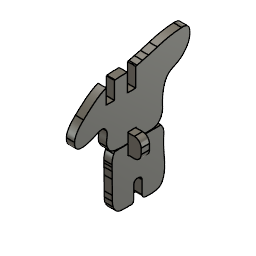
MORFY Test1 (Autodesk Fusion 360 design; units mm, degrees)
Autodesk Fusion 360 part; units mm, degrees
note: some values were not read from the file. Chosen so that the rebuilt part matches the saved one: that a step has no effect; which pieces of a blend or face edit are solid. Set by a fixed rule: which sketch regions a step uses.
sketch "Sketch7" plane through (0, 0, 0) normal (1, 0, 0) x (0, 0, -1)
  line L0 (0, 0) -> (80, 0)
  line L1 (80, 0) -> (80, 80)
  line L2 (80, 80) -> (0, 80)
  line L3 (0, 80) -> (0, 0)
  line L4 (34, 0) -> (46, 0)
  line L5 (46, 0) -> (46, 30)
  line L6 (46, 30) -> (34, 30)
  line L7 (34, 30) -> (34, 0)
  line L8 (25.6401, 80) -> (37.6401, 80)
  line L9 (37.6401, 80) -> (37.6401, 65)
  line L10 (37.6401, 65) -> (25.6401, 65)
  line L11 (25.6401, 65) -> (25.6401, 80)
  line L12 (-92.3642, 110) -> (183.4543, 110)
  line L13 (183.4543, 110) -> (183.4543, 204.562)
  line L14 (-92.3642, 204.562) -> (-92.3642, 110)
  line L15 (25.6401, 110) -> (37.6401, 110)
  line L16 (37.6401, 110) -> (37.6401, 125)
  line L17 (37.6401, 125) -> (25.6401, 125)
  line L18 (25.6401, 125) -> (25.6401, 110)
  line L19 (24.6547, 204.562) -> (36.6547, 204.562)
  line L20 (36.6547, 204.562) -> (36.6547, 174.562)
  line L21 (36.6547, 174.562) -> (24.6547, 174.562)
  line L22 (24.6547, 174.562) -> (24.6547, 204.562)
  line L23 (-6.0953, 204.562) -> (5.9047, 204.562)
  line L24 (5.9047, 204.562) -> (5.9047, 174.562)
  line L25 (5.9047, 174.562) -> (-6.0953, 174.562)
  line L26 (-6.0953, 174.562) -> (-6.0953, 204.562)
  spline S0 degree 3 poles (115.5, 205.2559) (115.6659, 197.3379) (111.8252, 191.1596) (109.8122, 188.2657) knots 0 0 0 0 1 1 1 1
  spline S1 degree 3 poles (109.8122, 188.2657) (98.6392, 172.2077) (87.6076, 176.7145) (80.9024, 164.5312) knots 0 0 0 0 1 1 1 1
  spline S2 degree 3 poles (80.9024, 164.5312) (74.7119, 153.2655) (75.727, 134.0915) (75.7904, 133.0545) knots 0 0 0 0 1 1 1 1
  spline S3 degree 3 poles (75.7904, 133.0545) (75.8978, 131.2756) (76.3565, 125.3731) (73.2991, 119.5316) knots 0 0 0 0 1 1 1 1
  spline S4 degree 3 poles (73.2991, 119.5316) (72.5427, 118.0871) (71.0421, 115.3006) (67.9603, 113.3119) knots 0 0 0 0 1 1 1 1
  spline S5 degree 3 poles (67.9603, 113.3119) (64.7418, 111.2354) (61.499, 111.1281) (58.0561, 111.0597) knots 0 0 0 0 1 1 1 1
  spline S6 degree 3 poles (58.0561, 111.0597) (49.4695, 110.8865) (42.9277, 110.9475) (39.9264, 110.9377) knots 0 0 0 0 1 1 1 1
  spline S7 degree 2 poles (39.9264, 110.9377) (27.9262, 110.9036) (20.4889, 110.5059) knots 0 0 0 1 1 1
  spline S8 degree 3 poles (20.4889, 110.5059) (17.9976, 110.3741) (13.2956, 110.091) (7.4053, 111.2379) knots 0 0 0 0 1 1 1 1
  spline S9 degree 3 poles (7.4053, 111.2379) (3.4206, 112.0187) (1.4808, 112.9459) (-0.0686, 114.1879) knots 0 0 0 0 1 1 1 1
  spline S10 degree 3 poles (-0.0686, 114.1879) (-2.5477, 116.1692) (-3.6189, 118.7069) (-4.5559, 121.0054) knots 0 0 0 0 1 1 1 1
  spline S11 degree 3 poles (-4.5559, 121.0054) (-8.072, 129.6262) (-2.2427, 134.6698) (-5.8223, 142.2779) knots 0 0 0 0 1 1 1 1
  spline S12 degree 3 poles (-5.8223, 142.2779) (-7.4059, 145.6476) (-9.3409, 146.5626) (-9.802, 146.7627) knots 0 0 0 0 1 1 1 1
  spline S13 degree 3 poles (-9.802, 146.7627) (-12.469, 147.9266) (-15.2165, 146.7749) (-18.3618, 145.4866) knots 0 0 0 0 1 1 1 1
  spline S14 degree 3 poles (-18.3618, 145.4866) (-23.1907, 143.5077) (-33.8025, 138.7276) (-40.0783, 138.5177) knots 0 0 0 0 1 1 1 1
  spline S15 degree 3 poles (-40.0783, 138.5177) (-45.7417, 138.3299) (-47.7962, 139.8647) (-48.3135, 140.2258) knots 0 0 0 0 1 1 1 1
  spline S16 degree 3 poles (-48.3135, 140.2258) (-51.4856, 142.4828) (-52.4372, 146.8408) (-52.1005, 150.7181) knots 0 0 0 0 1 1 1 1
  spline S17 degree 3 poles (-52.1005, 150.7181) (-51.4661, 158.0382) (-47.3887, 164.4727) (-38.9095, 172.359) knots 0 0 0 0 1 1 1 1
  spline S18 degree 3 poles (-38.9095, 172.359) (-25.0036, 185.323) (-12.4788, 196.9767) (6.8319, 199.8438) knots 0 0 0 0 1 1 1 1
  spline S19 degree 3 poles (6.8319, 199.8438) (17.8292, 201.4835) (23.7268, 199.1899) (38.6039, 202.462) knots 0 0 0 0 1 1 1 1
  spline S20 degree 3 poles (38.6039, 202.462) (45.0774, 203.8845) (48.2251, 205.2559) (55.4232, 206.7614) knots 0 0 0 0 1 1 1 1
  spline S21 degree 2 poles (55.4232, 206.7614) (62.0968, 208.8598) (68.1335, 210.685) knots 0 0 0 1 1 1
  spline S22 degree 2 poles (68.1335, 210.685) (85.6678, 216.446) (103.4778, 217.4562) knots 0 0 0 1 1 1
  spline S23 degree 3 poles (103.4778, 217.4562) (106.035, 217.6026) (109.0777, 217.6221) (111.713, 215.7481) knots 0 0 0 0 1 1 1 1
  spline S24 degree 3 poles (111.713, 215.7481) (115.4658, 213.0811) (115.4512, 207.569) (115.5, 205.2559) knots 0 0 0 0 1 1 1 1
  line L27 (183.4543, 204.562) -> (46.6766, 204.562)
  line L28 (36.6547, 204.562) -> (-92.3642, 204.562)
  line L29 (36.6547, 204.562) -> (118.2693, 237.026)
  line L30 (118.2693, 237.026) -> (183.4543, 204.562)
  dimension "d65" = 80
  dimension "d66" = 12
  dimension "d67" = 30
  dimension "d68" = 80
  dimension "d69" = 12
  dimension "d70" = 15
  dimension "d74" = 30
  dimension "d77" = 12
  dimension "d78" = 15
  dimension "d79" = 12
  dimension "d80" = 12
  dimension "d81" = 30
  dimension "d82" = 30
  dimension "d85" = 18.75
  constraint horizontal L0
  constraint vertical L1
  constraint horizontal L2
  constraint vertical L3
  constraint coincident L0.start L3.end
  constraint horizontal L4
  constraint vertical L5
  constraint horizontal L6
  constraint vertical L7
  constraint coincident L0 L4.start
  constraint midpoint L0 L4
  constraint horizontal L8
  constraint vertical L9
  constraint horizontal L10
  constraint vertical L11
  constraint coincident L2 L8.start
  constraint horizontal L12
  constraint vertical L13
  constraint horizontal L27
  constraint vertical L14
  constraint horizontal L15
  constraint vertical L16
  constraint horizontal L17
  constraint vertical L18
  constraint coincident L12 L15.start
  constraint horizontal L19
  constraint vertical L20
  constraint horizontal L21
  constraint vertical L22
  constraint coincident L19.start L28
  constraint horizontal L23
  constraint vertical L24
  constraint horizontal L25
  constraint vertical L26
  constraint coincident L23.start L28
  constraint collinear L11 L18
  constraint coincident S20 L27.end
  constraint collinear L27 L28
  measures "d65" distance of L0.end L1.end
  measures "d66" distance of L5.end L6.end
  measures "d67" distance of L4.end L5.end
  measures "d68" distance of L1.end L2.end
  measures "d69" distance of L9.end L10.end
  measures "d70" distance of L8.start L10.end
  measures "d74" distance of L2 L12
  measures "d77" distance of L16.end L17.end
  measures "d78" distance of L15.end L16.end
  measures "d79" distance of L24.end L25.end
  measures "d80" distance of L20.end L21.end
  measures "d81" distance of L23.start L25.end
  measures "d82" distance of L19.end L20.end
  measures "d85" distance of L22 L24
extrude "Extrude10" add sketch "Sketch7" along normal blind 12 contours L0 L1 L2 L3 L5 L6 L7 L9 L10 L11 makes body 1
extrude "Extrude11" add sketch "Sketch7" along normal blind 12 separate body contours L12 L14 L18 L26 S7 S8 S9 S10 S11 S12 S13 S14 S15 S16 S17 S18 L28 | L12 L13 L16 S0 S1 S2 S3 S4 S5 S6 S7 L27 | L16 L17 L18 L20 L21 L22 L24 L25 L26 S0 S1 S2 S3 S4 S5 S6 S7 S8 S9 S10 S11 S12 S13 S14 S15 S16 S17 S18 S19 S20 L27 | L22 L24 S18 S19 L28 | L20 S0 S19 S20 S21 S22 S23 S24 L27 L29 L30 | S0 S20 S21 S22 S23 S24 L27 makes body 2
extrude "Extrude14" cut sketch "Sketch7" along normal up to surface (12 mm away) contours L16 L17 L18 L20 L21 L22 L24 L25 L26 S0 S1 S2 S3 S4 S5 S6 S7 S8 S9 S10 S11 S12 S13 S14 S15 S16 S17 S18 S19 S20 L27 | S0 S20 S21 S22 S23 S24 L27 keep common part bodies 2
move_body "Move3" bodies 2 to x (1, 0, 0) y (0, 1, 0) z (0, 0, 1) at (0, -30, 0)
sketch "Sketch8" plane through (0, 0, 0) normal (0, 0, 1) x (1, 0, 0)
  line L0 (-19, 94) -> (31, 94)
  line L1 (31, 94) -> (31, 66)
  line L2 (31, 66) -> (-19, 66)
  line L3 (-19, 66) -> (-19, 94)
  line L4 (0, 95) -> (12, 95)
  line L5 (0, 65) -> (12, 65)
  line L6 (6, 95) -> (6, 65) construction
  line L7 (0, 80) -> (12, 80)
  line L8 (-19, 80) -> (31, 80) construction
  line L9 (6, 94) -> (6, 66) construction
  dimension "d90" = 30
  dimension "d91" = 28
  dimension "d93" = 50
  constraint horizontal L0
  constraint vertical L1
  constraint horizontal L2
  constraint vertical L3
  constraint midpoint L4 L6.start
  constraint midpoint L5 L6.end
  constraint midpoint L3 L8.start
  constraint midpoint L1 L8.end
  constraint collinear L7 L8
  constraint midpoint L0 L9.start
  constraint midpoint L2 L9.end
  constraint collinear L6 L9
  measures "d90" distance of L4 L5
  measures "d91" distance of L0.end L1.end
  measures "d93" distance of L1.end L2.end
extrude "Extrude12" add sketch "Sketch8" along normal blind 12 from surface at -37.6401 separate body makes body 3
fillet "Fillet5" [no effect]
sketch "Sketch9" plane through (0, 0, 0) normal (-1, 0, 0) x (0, 0, 1)
  line L0 (-80, 0) -> (-46, 0)
  line L1 (-46, 0) -> (-46, 30)
  line L2 (-46, 30) -> (-34, 30)
  line L3 (-34, 30) -> (-34, 0)
  line L4 (-34, 0) -> (0, 0)
  line L5 (0, 0) -> (0, 80)
  line L6 (0, 80) -> (-25.6401, 80)
  line L7 (-25.6401, 80) -> (-25.6401, 65)
  line L8 (-25.6401, 65) -> (-37.6401, 65)
  line L9 (-37.6401, 65) -> (-37.6401, 80)
  line L10 (-37.6401, 80) -> (-80, 80)
  line L11 (-80, 80) -> (-80, 0)
sketch "Sketch10" plane through (0, 0, 0) normal (-1, 0, 0) x (0, 0, 1)
  line L0 (-34, 0) -> (0, 0)
  line L1 (0, 0) -> (0, 80)
  line L2 (0, 80) -> (-25.6401, 80)
  line L3 (-25.6401, 80) -> (-25.6401, 65)
  line L4 (-25.6401, 65) -> (-37.6401, 65)
  line L5 (-37.6401, 65) -> (-37.6401, 80)
  line L6 (-37.6401, 80) -> (-80, 80)
  line L7 (-80, 80) -> (-80, 0)
  line L8 (-80, 0) -> (-46, 0)
  line L9 (-46, 0) -> (-46, 30)
  line L10 (-46, 30) -> (-34, 30)
  line L11 (-34, 30) -> (-34, 0)
  spline S0 degree 3 poles (-73.7036, 81.706) (-75.3725, 79.425) (-76.9127, 77.0041) (-77.8839, 74.3392) knots 0 0 0 0 1 1 1 1
  arc A0 (-78.9408, 68.1331) -> (-77.8839, 74.3392) centre (-61.374, 68.3344) cw
  spline S1 degree 3 poles (-78.9408, 68.1331) (-78.9137, 65.6625) (-78.6043, 63.1986) (-78.4891, 60.7302) knots 0 0 0 0 1 1 1 1
  spline S2 degree 3 poles (-78.4891, 60.7302) (-78.3988, 58.9235) (-78.3988, 57.1326) (-78.4394, 55.3327) knots 0 0 0 0 1 1 1 1
  spline S3 degree 3 poles (-78.4394, 55.3327) (-78.5614, 50.0842) (-78.7533, 44.8086) (-79.196, 39.576) knots 0 0 0 0 1 1 1 1
  spline S4 degree 3 poles (-79.196, 39.576) (-79.4376, 36.7033) (-79.8509, 33.851) (-79.9548, 30.9648) knots 0 0 0 0 1 1 1 1
  spline S5 degree 3 poles (-79.9548, 30.9648) (-80.1422, 25.8428) (-80.0587, 20.6146) (-79.0198, 15.5784) knots 0 0 0 0 1 1 1 1
  arc A1 (-77.3102, 9.8715) -> (-79.0198, 15.5784) centre (-45.9875, 22.3642) cw
  spline S6 degree 3 poles (-77.3102, 9.8715) (-76.3436, 7.4505) (-75.2325, 5.0634) (-73.2158, 3.3222) knots 0 0 0 0 1 1 1 1
  spline S7 degree 3 poles (-73.2158, 3.3222) (-71.5762, 1.913) (-69.6024, 1.118) (-67.5179, 0.5941) knots 0 0 0 0 1 1 1 1
  arc A2 (-58.5002, -0.5983) -> (-67.5179, 0.5941) centre (-57.5378, 41.3739) cw
  spline S8 degree 3 poles (-58.5002, -0.5983) (-55.964, -0.6706) (-53.4324, -0.4809) (-50.8985, -0.386) knots 0 0 0 0 1 1 1 1
  spline S9 degree 3 poles (-50.8985, -0.386) (-45.9459, -0.2008) (-40.9865, -0.1195) (-36.0271, -0.1015) knots 0 0 0 0 1 1 1 1
  spline S10 degree 3 poles (-36.0271, -0.1015) (-31.4674, -0.0834) (-26.9077, -0.1015) (-22.3458, -0.0473) knots 0 0 0 0 1 1 1 1
  spline S11 degree 3 poles (-22.3458, -0.0473) (-19.349, -0.0066) (-16.2188, -0.1579) (-13.2739, 0.5105) knots 0 0 0 0 1 1 1 1
  arc A3 (-6.1781, 4.9618) -> (-13.2739, 0.5105) centre (-16.1754, 13.0173) cw
  spline S12 degree 3 poles (-6.1781, 4.9618) (-2.9667, 8.9072) (-1.7088, 14.0224) (-1.7223, 19.0315) knots 0 0 0 0 1 1 1 1
  spline S13 degree 3 poles (-1.7223, 19.0315) (-1.7381, 25.0952) (-1.6387, 31.159) (-1.5755, 37.2227) knots 0 0 0 0 1 1 1 1
  line L12 (-1.5755, 37.2227) -> (-1.3632, 57.7853)
  spline S14 degree 3 poles (-1.3632, 57.7853) (-1.3452, 59.4271) (-1.3836, 61.078) (-1.2864, 62.7153) knots 0 0 0 0 1 1 1 1
  spline S15 degree 3 poles (-1.2864, 62.7153) (-1.2187, 63.8445) (-1.1938, 64.9985) (-1.2187, 66.139) knots 0 0 0 0 1 1 1 1
  arc A4 (-1.9888, 72.7448) -> (-1.2187, 66.139) centre (-34.5458, 65.6015) cw
  spline S16 degree 3 poles (-1.9888, 72.7448) (-2.8989, 76.8211) (-4.8231, 80.7755) (-8.0684, 83.5082) knots 0 0 0 0 1 1 1 1
  arc A5 (-13.9017, 86.7015) -> (-8.0684, 83.5082) centre (-19.127, 70.2317) cw
  arc A6 (-17.8675, 87.6433) -> (-13.9017, 86.7015) centre (-23.2006, 56.3645) cw
  arc A7 (-22.7636, 88.2463) -> (-17.8675, 87.6433) centre (-25.5631, 45.3357) cw
  spline S17 degree 3 poles (-22.7636, 88.2463) (-25.9728, 88.4721) (-29.1887, 88.4427) (-32.4024, 88.4721) knots 0 0 0 0 1 1 1 1
  spline S18 degree 3 poles (-32.4024, 88.4721) (-35.3609, 88.4992) (-38.3193, 88.5647) (-41.2778, 88.6189) knots 0 0 0 0 1 1 1 1
  spline S19 degree 3 poles (-41.2778, 88.6189) (-46.4111, 88.7137) (-51.5715, 88.8199) (-56.689, 88.3366) knots 0 0 0 0 1 1 1 1
  spline S20 degree 3 poles (-56.689, 88.3366) (-60.9054, 87.9369) (-65.1669, 87.1193) (-68.961, 85.15) knots 0 0 0 0 1 1 1 1
  arc A8 (-73.6133, 81.8212) -> (-68.961, 85.15) centre (-59.5693, 67.1093) cw
  spline S21 degree 3 poles (-73.6133, 81.8212) (-74.1327, 81.3176) (-73.3332, 80.5204) (-72.8002, 81.024) knots 0 0 0 0 1 1 1 1
  spline S22 degree 3 poles (-72.8002, 81.024) (-69.966, 83.7363) (-66.3774, 85.3601) (-62.5879, 86.2634) knots 0 0 0 0 1 1 1 1
  spline S23 degree 3 poles (-62.5879, 86.2634) (-58.1343, 87.3248) (-53.5069, 87.51) (-48.9473, 87.5484) knots 0 0 0 0 1 1 1 1
  spline S24 degree 3 poles (-48.9473, 87.5484) (-43.3781, 87.5959) (-37.8134, 87.3813) (-32.2465, 87.3361) knots 0 0 0 0 1 1 1 1
  spline S25 degree 3 poles (-32.2465, 87.3361) (-29.0555, 87.309) (-25.8644, 87.3361) (-22.6801, 87.1103) knots 0 0 0 0 1 1 1 1
  arc A9 (-22.6801, 87.1103) -> (-17.9217, 86.5073) centre (-25.2821, 47.5002) cw
  arc A10 (-17.9217, 86.5073) -> (-14.0824, 85.5859) centre (-23.408, 55.1885) cw
  arc A11 (-14.0824, 85.5859) -> (-4.9315, 77.7267) centre (-19.0277, 70.5707) cw
  spline S26 degree 3 poles (-4.9315, 77.7267) (-2.9825, 73.9507) (-2.3411, 69.5966) (-2.3276, 65.3915) knots 0 0 0 0 1 1 1 1
  spline S27 degree 3 poles (-2.3276, 65.3915) (-2.3276, 64.2239) (-2.4247, 63.0653) (-2.4382, 61.9023) knots 0 0 0 0 1 1 1 1
  line L13 (-2.4382, 61.9023) -> (-2.4902, 56.8255)
  line L14 (-2.4902, 56.8255) -> (-2.594, 46.7644)
  line L15 (-2.594, 46.7644) -> (-2.8041, 26.5496)
  spline S28 degree 2 poles (-2.8041, 26.5496) (-2.8447, 22.742) (-2.8402, 18.9366) knots 0 0 0 1 1 1
  arc A12 (-2.8402, 18.9366) -> (-3.9423, 11.4366) centre (-26.4737, 18.5784) cw
  spline S29 degree 3 poles (-3.9423, 11.4366) (-4.6672, 9.2527) (-5.8009, 7.0621) (-7.3299, 5.3389) knots 0 0 0 0 1 1 1 1
  arc A13 (-7.3299, 5.3389) -> (-14.6267, 1.4229) centre (-16.298, 13.2933) cw
  arc A14 (-14.6267, 1.4229) -> (-18.886, 1.1632) centre (-18.7684, 34.2912) cw
  spline S30 degree 2 poles (-18.886, 1.1632) (-21.2799, 1.1158) (-23.6783, 1.0909) knots 0 0 0 1 1 1
  spline S31 degree 2 poles (-23.6783, 1.0909) (-27.504, 1.048) (-31.3274, 1.0525) knots 0 0 0 1 1 1
  spline S32 degree 3 poles (-31.3274, 1.0525) (-36.07, 1.0525) (-40.8126, 1.0367) (-45.5552, 0.9261) knots 0 0 0 0 1 1 1 1
  spline S33 degree 3 poles (-45.5552, 0.9261) (-48.1884, 0.8651) (-50.824, 0.7928) (-53.4595, 0.6573) knots 0 0 0 0 1 1 1 1
  spline S34 degree 3 poles (-53.4595, 0.6573) (-58.2021, 0.4134) (-62.9447, 0.5692) (-67.5563, 1.7978) knots 0 0 0 0 1 1 1 1
  spline S35 degree 3 poles (-67.5563, 1.7978) (-69.6024, 2.3421) (-71.5017, 3.1822) (-73.0125, 4.7021) knots 0 0 0 0 1 1 1 1
  spline S36 degree 3 poles (-73.0125, 4.7021) (-74.7108, 6.4117) (-75.6706, 8.6949) (-76.4995, 10.9194) knots 0 0 0 0 1 1 1 1
  spline S37 degree 3 poles (-76.4995, 10.9194) (-78.0555, 15.0906) (-78.6494, 19.5012) (-78.8233, 23.9389) knots 0 0 0 0 1 1 1 1
  arc A15 (-78.8233, 23.9389) -> (-78.4733, 35.5922) centre (-0.7613, 27.4259) cw
  spline S38 degree 3 poles (-78.4733, 35.5922) (-78.0013, 39.8176) (-77.7529, 44.0453) (-77.5699, 48.2933) knots 0 0 0 0 1 1 1 1
  spline S39 degree 3 poles (-77.5699, 48.2933) (-77.387, 52.5413) (-77.1499, 56.7645) (-77.3712, 60.9967) knots 0 0 0 0 1 1 1 1
  spline S40 degree 3 poles (-77.3712, 60.9967) (-77.4977, 63.3973) (-77.798, 65.798) (-77.8229, 68.2009) knots 0 0 0 0 1 1 1 1
  arc A16 (-77.8229, 68.2009) -> (-76.7524, 74.154) centre (-61.1833, 68.2816) cw
  spline S41 degree 3 poles (-76.7524, 74.154) (-75.8152, 76.6834) (-74.3088, 78.9756) (-72.7189, 81.1369) knots 0 0 0 0 1 1 1 1
  spline S42 degree 3 poles (-72.7189, 81.1369) (-72.2876, 81.7241) (-73.2677, 82.2864) (-73.7036, 81.706) knots 0 0 0 0 1 1 1 1
extrude "Extrude13" cut sketch "Sketch10" against normal up to surface (12 mm away) contours L2 L3 L4 L5 L6 L9 L10 L11 A11 S26 S27 L13 L14 L15 S28 A12 S29 A13 A14 S30 S31 S32 S33 S34 S35 S36 S37 A15 S38 S39 S40 A16 S41 keep common part bodies 1
fillet "Fillet7" radius 5 2 edges at (6, 30, -34) (6, 30, -46) on bodies 1
fillet "Fillet9" radius 5 2 edges at (6, 0.9157, -46) (6, 1.0503, -34) on bodies 1
fillet "Fillet10" radius 10 4 edges at (-19, 94, -31.6401) (-19, 66, -31.6401) (31, 94, -31.6401) (31, 66, -31.6401) on bodies 3
equation "esp = 12 mm"
equation "slot = 30 mm"
equation "distance = 30 mm"
equation "plus = 2 mm"
equation "freza = 6 mm"
equation "fillet = 5 mm"
equation "alt = 80 mm"
equation "d65 = alt"
equation "d66 = esp"
equation "d67 = slot"
equation "d68 = alt"
equation "d69 = esp"
equation "d70 = slot / 2"
equation "d74 = distance"
equation "d77 = esp"
equation "d78 = d70"
equation "d79 = esp"
equation "d80 = esp"
equation "d81 = slot"
equation "d82 = slot"
equation "d83 = 150.00 mm"
equation "d85 = d83 / 8"
equation "d86 = esp"
equation "d88 = esp"
equation "d91 = d90 - plus"
equation "d92 = slot * 2"
equation "d96 = esp"
equation "d103 = fillet"
equation "d109 = fillet"
